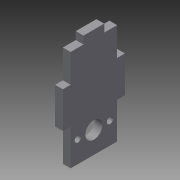
# Autodesk Inventor part: AngleLower
Saved by Autodesk Inventor 2013 (Build 170138000, 138)
## iProperties
Created: 2013-04-21
Part Number: AngleLower
Material: Generic
Document SubType Name: Modeling
Designer: fuji
Density: 1 g/cm^3
Author: fuji
Autodesk Inventor part; units mm, degrees
ref_plane "YZ Plane" through (0, 0, 0) normal (1, 0, 0) x (0, 1, 0)
ref_plane "XZ Plane" through (0, 0, 0) normal (0, 1, 0) x (-1, 0, 0)
ref_plane "XY Plane" through (0, 0, 0) normal (0, 0, 1) x (1, 0, 0)
sketch "Sketch1" plane through (0, 0, 0) normal (1, 0, 0) x (0, 1, 0)
  line L0 (0, 0) -> (41.275, 0)
  line L1 (41.275, 0) -> (41.275, -19.05)
  line L2 (41.275, -19.05) -> (0, -19.05)
  line L3 (0, -19.05) -> (0, 0)
  dimension "d0" = 41.275
  dimension "d1" = 19.05
  constraints: 8 end point, 2 parallel, 1 horizontal, 1 perpendicular
  measures "d0" distance of L1.end L2.end
  measures "d1" distance of L0.end L1.end
extrude "Extrusion1" add sketch "Sketch1" along normal blind 3.175
sketch "Sketch2" plane through (3.175, 0, 0) normal (1, 0, 0) x (0, 0, -1)
  line L0 (0, 41.275) -> (0, 0) projected
  line L1 (0, 0) -> (19.05, 0) projected
  line L2 (19.05, 0) -> (19.05, 41.275) projected
  line L3 (19.05, 41.275) -> (0, 41.275) projected
  line L4 (5.2917, 41.275) -> (13.7583, 41.275)
  line L5 (13.7583, 41.275) -> (13.7583, 44.45)
  line L6 (13.7583, 44.45) -> (5.2917, 44.45)
  line L7 (5.2917, 44.45) -> (5.2917, 41.275)
  line L8 (19.05, 29.6333) -> (22.225, 29.6333)
  line L9 (22.225, 29.6333) -> (22.225, 14.8167)
  line L10 (22.225, 14.8167) -> (19.05, 14.8167)
  line L11 (19.05, 14.8167) -> (19.05, 29.6333)
  line L12 (0, 29.6333) -> (-3.175, 29.6333)
  line L13 (-3.175, 29.6333) -> (-3.175, 14.8167)
  line L14 (-3.175, 14.8167) -> (0, 14.8167)
  line L15 (0, 14.8167) -> (0, 29.6333)
  dimension "d4" = 8.4667
  dimension "d5" = 3.175
  dimension "d6" = 5.2917
  dimension "d7" = 3.175
  dimension "d8" = 14.8167
  dimension "d9" = 3.175
  dimension "d10" = 14.8167
  dimension "d11" = 14.8167
  constraints: 24 end point, 6 parallel, 3 horizontal, 3 perpendicular, 3 point on line, 1 collinear
  measures "d4" distance of L6.end L5.end
  measures "d5" distance of L5.end L4.end
  measures "d6" distance between parallel lines of L7 L0
  measures "d7" distance of L9.end L10.end
  measures "d8" distance of L8.end L9.end
  measures "d9" distance of L14.end L13.end
  measures "d10" distance of L13.end L12.end
  measures "d11" distance between parallel lines of L14 L1
extrude "Extrusion2" add sketch "Sketch2" against normal blind 3.175 contours L0 L14 L13 L12 | L7 L6 L5 L3 | L8 L9 L10 L2
sketch "Sketch3" plane through (3.175, 0, 0) normal (1, 0, 0) x (0, 0, -1)
  line L0 (-3.175, 29.6333) -> (-3.175, 14.8167) projected
  line L1 (0, 0) -> (19.05, 0) projected
  circle A0 centre (9.525, 8.89) radius 3.5052
  circle A1 centre (16.1036, 8.89) radius 0.889
  circle A2 centre (2.9464, 8.89) radius 0.889
  dimension "d14" = 7.0104
  dimension "d15" = 12.7
  dimension "d16" = 8.89
  dimension "d17" = 1.778
  dimension "d18" = 1.778
  dimension "d19" = 13.1572
  dimension "d20" = 6.5786
  constraints: 3 centre point
  measures "d14" diameter of A0
  measures "d15" distance from line of A0.centre L0
  measures "d16" distance from line of L1 A0.centre
  measures "d17" diameter of A1
  measures "d18" diameter of A2
  measures "d19" distance of A1.centre A2.centre
  measures "d20" distance of A0.centre A1.centre
extrude "Extrusion3" cut sketch "Sketch3" against normal blind 3.175
equation "\"d0\" = angleHeight - thick"
equation "\"d1\" = angleDepth - 2 * thick"
equation "\"d2\" = thick"
equation "\"d4\" = 0.333333 * angleDepth"
equation "\"d5\" = thick"
equation "\"d6\" = 0.333333 * angleDepth - thick"
equation "\"d7\" = thick"
equation "\"d8\" = 0.333333 * angleHeight"
equation "\"d9\" = thick"
equation "\"d10\" = 0.333333 * angleHeight"
equation "\"d11\" = 0.333333 * angleHeight"
equation "\"d12\" = thick"
equation "\"d14\" = hornCenter"
equation "\"d15\" = 0.5 * angleDepth"
equation "\"d16\" = hornOffset"
equation "\"d17\" = hornHole"
equation "\"d18\" = hornHole"
equation "\"d19\" = hornDia"
equation "\"d20\" = 0.5 * hornDia"
equation "\"d21\" = thick"
equation "\"angleHeight\" = 44.45"
equation "\"angleDepth\" = 25.4"
equation "\"hornCenter\" = 7.0104"
equation "\"hornOffset\" = 8.89"
equation "\"thick\" = 3.175"
equation "\"hornHole\" = 1.778"
equation "\"hornDia\" = 13.1572"
body "Solid1"
